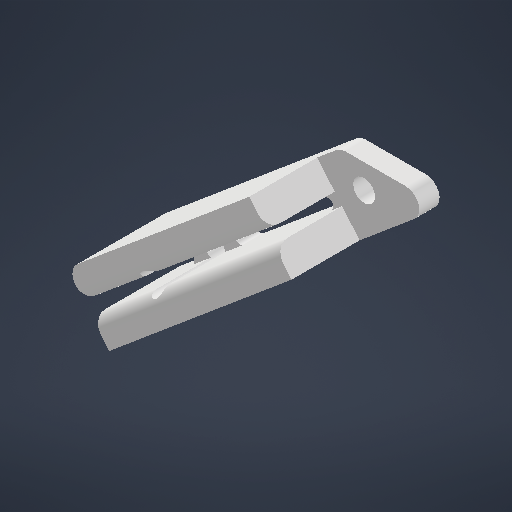
# Autodesk Inventor part: rpi-mount-clip
Saved by Autodesk Inventor 2025 (Build 290162000, 162)
## iProperties
Created: 2024-10-27
Part Number: rpi-mount-clip
Material: Generic
Document SubType Name: Modeling
Designer: Windows 7 was better
Density: 1 g/cm^3
Appearance: Default
Author: Windows 7 was better
Autodesk Inventor part; units mm, degrees
ref_plane "YZ Plane" through (0, 0, 0) normal (1, 0, 0) x (0, 1, 0)
ref_plane "XZ Plane" through (0, 0, 0) normal (0, 1, 0) x (-1, 0, 0)
ref_plane "XY Plane" through (0, 0, 0) normal (0, 0, 1) x (1, 0, 0)
sketch "Sketch1" plane through (0, 0, 0) normal (0, 0, 1) x (1, 0, 0)
  arc A0 (-5.9347, 9.1506) -> (-6.1812, 6.3329) centre (-4.6492, 7.6185) ccw projected
  line L0 (-4.8957, 4.8008) -> (-6.1812, 6.3329) projected
  line L1 (1.2318, 9.9424) -> (-4.8957, 4.8008) projected
  line L2 (1.2318, 7.7232) -> (1.2318, 9.9424) projected
  line L3 (-3.8029, 3.4986) -> (1.2318, 7.7232) projected
  line L4 (0.7639, -1.9439) -> (-3.8029, 3.4986) projected
  arc A1 (1.2318, -3.2295) -> (0.7639, -1.9439) centre (-0.7682, -3.2295) ccw projected
  line L5 (1.2318, -14.0349) -> (1.2318, -3.2295) projected
  arc A2 (-0.0682, -15.9084) -> (1.2318, -14.0349) centre (-0.7682, -14.0349) ccw projected
  arc A3 (-0.0682, -15.9084) -> (-1.3682, -17.7819) centre (0.6318, -17.7819) ccw projected
  line L6 (-1.3682, -20.9819) -> (-1.3682, -17.7819) projected
  arc A4 (-1.3682, -20.9819) -> (0.6318, -22.9819) centre (0.6318, -20.9819) ccw projected
  line L7 (65.8318, -22.9819) -> (0.6318, -22.9819) projected
  arc A5 (65.8318, -22.9819) -> (67.8318, -20.9819) centre (65.8318, -20.9819) ccw projected
  line L8 (67.8318, -16.9174) -> (67.8318, -20.9819) projected
  arc A6 (67.8318, -16.9174) -> (67.1285, -15.3947) centre (65.8318, -16.9174) ccw projected
  arc A7 (66.4252, -13.872) -> (67.1285, -15.3947) centre (68.4252, -13.872) ccw projected
  line L9 (66.4252, 24.1081) -> (66.4252, -13.872) projected
  arc A8 (67.1285, 25.6308) -> (66.4252, 24.1081) centre (68.4252, 24.1081) ccw projected
  arc A9 (67.1285, 25.6308) -> (67.8318, 27.1535) centre (65.8318, 27.1535) ccw projected
  line L10 (67.8318, 31.2181) -> (67.8318, 27.1535) projected
  arc A10 (67.8318, 31.2181) -> (65.8318, 33.2181) centre (65.8318, 31.2181) ccw projected
  line L11 (0.6318, 33.2181) -> (65.8318, 33.2181) projected
  arc A11 (0.6318, 33.2181) -> (-1.3682, 31.2181) centre (0.6318, 31.2181) ccw projected
  line L12 (-1.3682, 28.0181) -> (-1.3682, 31.2181) projected
  arc A12 (-1.3682, 28.0181) -> (-0.0682, 26.1446) centre (0.6318, 28.0181) ccw projected
  arc A13 (1.2318, 24.2711) -> (-0.0682, 26.1446) centre (-0.7682, 24.2711) ccw projected
  line L13 (1.2318, 16.0966) -> (1.2318, 24.2711) projected
  arc A14 (0.5174, 14.5645) -> (1.2318, 16.0966) centre (-0.7682, 16.0966) ccw projected
  line L14 (-5.9347, 9.1506) -> (0.5174, 14.5645) projected
  arc A15 (20.663, 26.0181) -> (20.1809, 25.8426) centre (20.663, 25.2681) ccw projected
  line L15 (20.9741, 26.0181) -> (20.663, 26.0181) projected
  arc A16 (21.4562, 24.6935) -> (20.9741, 26.0181) centre (20.9741, 25.2681) ccw projected
  line L16 (8.4639, 13.7916) -> (21.4562, 24.6935) projected
  arc A17 (7.2318, 14.3662) -> (8.4639, 13.7916) centre (7.9818, 14.3662) ccw projected
  line L17 (7.2318, 14.6273) -> (7.2318, 14.3662) projected
  arc A18 (7.4997, 15.2018) -> (7.2318, 14.6273) centre (7.9818, 14.6273) ccw projected
  line L18 (20.1809, 25.8426) -> (7.4997, 15.2018) projected
  circle A19 centre (4.2318, 29.6181) radius 1.1 projected
  circle A20 centre (62.2318, 29.6181) radius 1.1 projected
  circle A21 centre (26.2369, 29.6181) radius 1.6 projected
  circle A22 centre (4.2318, -19.3819) radius 1.1 projected
  circle A23 centre (62.2318, -19.3819) radius 1.1 projected
  arc A24 (58.4252, -15.7819) -> (60.4252, -13.7819) centre (58.4252, -13.7819) ccw projected
  line L19 (39.4252, -15.7819) -> (58.4252, -15.7819) projected
  arc A25 (37.4252, -13.7819) -> (39.4252, -15.7819) centre (39.4252, -13.7819) ccw projected
  line L20 (37.4252, 24.0181) -> (37.4252, -13.7819) projected
  arc A26 (39.4252, 26.0181) -> (37.4252, 24.0181) centre (39.4252, 24.0181) ccw projected
  line L21 (58.4252, 26.0181) -> (39.4252, 26.0181) projected
  arc A27 (60.4252, 24.0181) -> (58.4252, 26.0181) centre (58.4252, 24.0181) ccw projected
  line L22 (60.4252, -13.7819) -> (60.4252, 24.0181) projected
  circle A28 centre (4.2318, 11.3501) radius 1.6 projected
  arc A29 (31.4252, 23.5479) -> (28.1396, 25.0799) centre (29.4252, 23.5479) ccw projected
  line L23 (31.4252, -13.7819) -> (31.4252, 23.5479) projected
  arc A30 (29.4252, -15.7819) -> (31.4252, -13.7819) centre (29.4252, -13.7819) ccw projected
  line L24 (7.2318, -15.7819) -> (29.4252, -15.7819) projected
  line L25 (7.2318, 6.6036) -> (7.2318, -15.7819) projected
  arc A31 (7.9462, 8.1356) -> (7.2318, 6.6036) centre (9.2318, 6.6036) ccw projected
  line L26 (28.1396, 25.0799) -> (7.9462, 8.1356) projected
  arc A32 (12.5886, 24.6935) -> (12.1065, 26.0181) centre (12.1065, 25.2681) ccw projected
  line L27 (8.4639, 21.2325) -> (12.5886, 24.6935) projected
  arc A33 (7.2318, 21.807) -> (8.4639, 21.2325) centre (7.9818, 21.807) ccw projected
  line L28 (7.2318, 25.2681) -> (7.2318, 21.807) projected
  arc A34 (7.9818, 26.0181) -> (7.2318, 25.2681) centre (7.9818, 25.2681) ccw projected
  line L29 (12.1065, 26.0181) -> (7.9818, 26.0181) projected
  line L30 (7.9462, 8.1356) -> (-1.2318, 0.4344)
  line L31 (-1.2318, 0.4344) -> (25.5798, 22.932) construction
  line L32 (25.5798, 22.932) -> (19.3447, 30.3626) construction
  line L33 (19.3447, 30.3626) -> (-7.4668, 7.865) construction
  line L34 (-7.4668, 7.865) -> (-1.2318, 0.4344) construction
  line L35 (25.5798, 22.932) -> (28.1396, 25.0799)
  line L36 (21.9046, 32.5106) -> (-5.9347, 9.1506)
  line L37 (7.9462, 8.1356) -> (37.8383, 33.2181)
  line L38 (21.9046, 32.5106) -> (22.7477, 33.2181)
  point P0 (0, 0)
  point P1 (28.1396, 25.0799)
  point P2 (12.5886, 24.6935)
  point P3 (0.5174, 14.5645)
  dimension "d0" = 35
  constraints: 18 end point, 8 point on line, 2 perpendicular, 1 collinear, 1 parallel, 1 point on circle
  measures "d0" distance of L30.end L31.end
extrude "Extrusion1" add sketch "Sketch1" along normal blind 3 contours L14 L36 L27 L38 L11 L37 L26 L30 L4 L3 L2 L1 L0 A0
fillet "Fillet1" radius 2 2 edges at (37.8383, 33.2181, 1.5) (22.7477, 33.2181, 1.5)
sketch "Sketch2" plane through (0, 0, 3) normal (0, 0, 1) x (1, 0, 0)
  arc A0 (23.4757, 33.2181) -> (22.1901, 32.7501) centre (23.4757, 31.2181) ccw projected
  line L0 (22.1901, 32.7501) -> (-5.9347, 9.1506) projected
  arc A1 (-5.9347, 9.1506) -> (-6.1812, 6.3329) centre (-4.6492, 7.6185) ccw projected
  line L1 (-6.1812, 6.3329) -> (-4.8957, 4.8008) projected
  line L2 (-4.8957, 4.8008) -> (1.2318, 9.9424) projected
  line L3 (1.2318, 9.9424) -> (1.2318, 7.7232) projected
  line L4 (1.2318, 7.7232) -> (-3.8029, 3.4986) projected
  line L5 (-3.8029, 3.4986) -> (-1.2318, 0.4344) projected
  line L6 (-1.2318, 0.4344) -> (33.6289, 29.686) projected
  arc A2 (33.6289, 29.686) -> (32.3433, 33.2181) centre (32.3433, 31.2181) ccw projected
  line L7 (32.3433, 33.2181) -> (23.4757, 33.2181) projected
  circle A3 centre (4.2318, 11.3501) radius 1.6 projected
  circle A4 centre (26.2369, 29.6181) radius 1.6 projected
  line L8 (20.663, 26.0181) -> (20.9741, 26.0181) projected
  arc A5 (21.4562, 24.6935) -> (20.9741, 26.0181) centre (20.9741, 25.2681) ccw projected
  line L9 (21.4562, 24.6935) -> (8.4639, 13.7916) projected
  arc A6 (7.2318, 14.3662) -> (8.4639, 13.7916) centre (7.9818, 14.3662) ccw projected
  line L10 (7.2318, 14.3662) -> (7.2318, 14.6273) projected
  arc A7 (7.4997, 15.2018) -> (7.2318, 14.6273) centre (7.9818, 14.6273) ccw projected
  line L11 (7.4997, 15.2018) -> (20.1809, 25.8426) projected
  arc A8 (20.663, 26.0181) -> (20.1809, 25.8426) centre (20.663, 25.2681) ccw projected
  line L12 (-4.8957, 4.8008) -> (28.9706, 33.2181)
  line L13 (-1.2318, 0.4344) -> (25.5798, 22.932)
  line L14 (25.5798, 22.932) -> (21.9159, 27.2984)
  line L15 (-3.8029, 3.4986) -> (23.0086, 25.9961)
  line L16 (21.9159, 27.2984) -> (19.3447, 30.3626)
  point P0 (0, 0)
  point P1 (21.4562, 24.6935)
  point P2 (8.4639, 13.7916)
  point P3 (5.8166, 11.5703)
  point P4 (3.7397, 9.8276)
  point P5 (2.647, 11.1299)
  point P6 (4.7238, 12.8726)
  point P7 (7.4997, 15.2018)
  dimension "d4" = 35
  constraints: 10 end point, 7 point on line, 2 perpendicular
  measures "d4" distance of L5.end L13.end
extrude "Extrusion2" add sketch "Sketch2" along normal blind 10 contours L16 L12 L11 A3 L2 L1 A1 L0 | L14 L6 L5 L4 L15 A3 L9
fillet "Fillet2" radius 2 3 edges at (13.3199, 20.0855, 13) (15.7362, 19.8939, 13) (7.1402, 12.681, 13)
body "Solid1"
